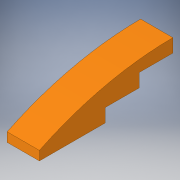
# Autodesk Inventor part: 3x1 curve
Saved by Autodesk Inventor 2017 (Build 210142000, 142)
## iProperties
Created: 2018-05-14
Part Number: 3x1 curve
Material: ABS Plastic
Document SubType Name: Modeling
Designer: 20000650
Density: 1.06 g/cm^3
Appearance: Orange
Author: 20000650
Autodesk Inventor part; units mm, degrees
ref_plane "YZ Plane" through (0, 0, 0) normal (1, 0, 0) x (0, 1, 0)
ref_plane "XZ Plane" through (0, 0, 0) normal (0, 1, 0) x (-1, 0, 0)
ref_plane "XY Plane" through (0, 0, 0) normal (0, 0, 1) x (1, 0, 0)
sketch "Sketch1" plane through (0, 0, 0) normal (1, 0, 0) x (0, 1, 0)
  line L0 (0, 0) -> (0, -15.9233)
  line L1 (0, -15.9233) -> (3.236, -15.9233)
  line L2 (3.236, -15.9233) -> (3.236, -24.1071)
  line L3 (3.236, -24.1071) -> (6.4618, -24.1071)
  line L4 (6.4618, -24.1071) -> (6.4618, -32.2859)
  line L5 (6.4618, -32.2859) -> (9.6876, -32.2859)
  line L6 (0, 0) -> (2.2149, 0)
  line L7 (9.6876, -32.2859) -> (40.3351, -32.2859) construction
  arc A0 (9.6876, -32.2859) -> (2.2149, 0) centre (-65.2438, -32.6213) ccw
  dimension "d0" = 15.9233
  dimension "d1" = 3.236
  dimension "d2" = 3.2258
  dimension "d3" = 3.2258
  dimension "d4" = 24.1071
  dimension "d5" = 32.2859
  dimension "d6" = 2.2149
  constraints: 16 end point, 5 perpendicular, 2 horizontal, 2 point on circle, 1 centre point, 1 vertical
  measures "d0" distance of L0.start L0.end
  measures "d1" distance of L0.end L1.end
  measures "d2" distance of L2.end L3.end
  measures "d3" distance of L4.end L5.end
  measures "d4" vertical distance of L2.end L0.start
  measures "d5" vertical distance of L0.start L4.end
  measures "d6" distance of L0.start L6.end
extrude "Extrusion1" add sketch "Sketch1" along normal blind 7.7978
shell "Shell1" thickness 1.4732 removed faces 3 at (2.5993, 0, -5.3078) at (2.5993, 3.236, -18.6512) at (2.5993, 6.4618, -26.8334)
sketch "Sketch5" plane through (0, 3.236, -24.1071) normal (0, -1, 0) x (1, 0, 0)
  line L0 (6.3246, 8.1839) -> (7.7978, 8.1839) projected
  line L1 (7.7978, 8.1839) -> (1.4732, 8.1839)
  line L2 (1.4732, 8.1839) -> (1.4732, 9.6571)
  line L3 (1.4732, 9.6571) -> (7.7978, 9.6571)
  line L4 (7.7978, 9.6571) -> (7.7978, 8.1839)
  line L5 (0, 8.1839) -> (1.4732, 8.1839) projected
  line L6 (1.4732, 9.6571) -> (0, 9.6571)
  line L7 (0, 9.6571) -> (0, 8.1839)
  line L8 (0, 8.1839) -> (1.4732, 8.1839)
  line L9 (1.4732, 8.1839) -> (1.4732, 9.6571)
  point P0 (0, 24.1071)
  constraints: 16 end point, 4 parallel, 2 horizontal, 2 perpendicular
extrude "Extrusion2" add sketch "Sketch5" against normal up to surface round surface about axis through (0, -65.2438, -32.6213) along (1, 0, 0) radius 73.4589 far side no
sketch "Sketch8" plane through (0, 3.236, -24.1071) normal (0, -1, 0) x (1, 0, 0)
  line L0 (1.4732, 1.4732) -> (6.3246, 1.4732) projected
  line L1 (6.3246, 1.4732) -> (1.4732, 1.4732)
  line L2 (1.4732, 1.4732) -> (1.4732, 0)
  line L3 (1.4732, 0) -> (6.3246, 0)
  line L4 (6.3246, 0) -> (6.3246, 1.4732)
  point P0 (0, 24.1071)
  point P1 (7.7978, 0)
  point P2 (0, 0)
  constraints: 8 end point, 3 equal length, 1 perpendicular
extrude "Extrusion3" add sketch "Sketch8" against normal up to surface round surface about axis through (0, -65.2438, -32.6213) along (1, 0, 0) radius 73.4589 far side no
sketch "Sketch9" plane through (0, 0, -15.9233) normal (0, -1, 0) x (1, 0, 0)
  line L0 (1.4732, -6.7107) -> (1.4732, 0) projected
  line L1 (6.3246, 1.4732) -> (1.4732, 1.4732) projected
  line L2 (1.4732, 1.4732) -> (1.4732, 14.4501) projected
  line L3 (1.4732, 14.4501) -> (6.3246, 14.4501) projected
  line L4 (6.3246, 14.4501) -> (6.3246, 1.4732) projected
  line L5 (0, 15.9233) -> (0, 0) projected
  line L6 (0, 0) -> (7.7978, 0) projected
  line L7 (7.7978, 15.9233) -> (7.7978, 0) projected
  line L8 (0, 15.9233) -> (7.7978, 15.9233) projected
  line L9 (0, -8.1839) -> (7.7978, -8.1839) projected
  line L10 (7.7978, 0) -> (7.7978, -8.1839) projected
  line L11 (6.3246, 0) -> (7.7978, 0) projected
  line L12 (6.3246, 0) -> (6.3246, -6.7107) projected
  line L13 (6.3246, -6.7107) -> (1.4732, -6.7107) projected
  line L14 (1.4732, -6.7107) -> (1.4732, 0) projected
  line L15 (0, 0) -> (1.4732, 0) projected
  line L16 (0, 0) -> (0, -8.1839) projected
  line L17 (1.4732, -14.8895) -> (1.4732, -8.1839) projected
  line L18 (0, -8.1839) -> (1.4732, -8.1839) projected
  line L19 (0, -8.1839) -> (0, -16.3627) projected
  line L20 (0, -16.3627) -> (7.7978, -16.3627) projected
  line L21 (7.7978, -8.1839) -> (7.7978, -16.3627) projected
  line L22 (6.3246, -8.1839) -> (7.7978, -8.1839) projected
  line L23 (6.3246, -8.1839) -> (6.3246, -14.8895) projected
  line L24 (6.3246, -14.8895) -> (1.4732, -14.8895) projected
  line L25 (6.3246, 0) -> (1.4732, 0) projected
  line L26 (6.3246, -6.7107) -> (1.4732, -6.7107) projected
  line L27 (4.5491, -1.7297) -> (3.2487, -1.7297)
  line L28 (3.2487, 0) -> (3.2487, -1.7297)
  line L29 (4.5491, -1.7297) -> (4.5491, 0)
  line L30 (4.5491, 0) -> (3.2487, 0)
  constraints: 8 end point, 2 point on line, 1 collinear, 1 parallel, 1 perpendicular
extrude "Extrusion4" add sketch "Sketch9" against normal up to surface from surface at -3.236 contours L6 L29 L27 L28 round surface about axis through (0, -65.2438, -32.6213) along (1, 0, 0) radius 73.4589 far side no
body "Solid1"
